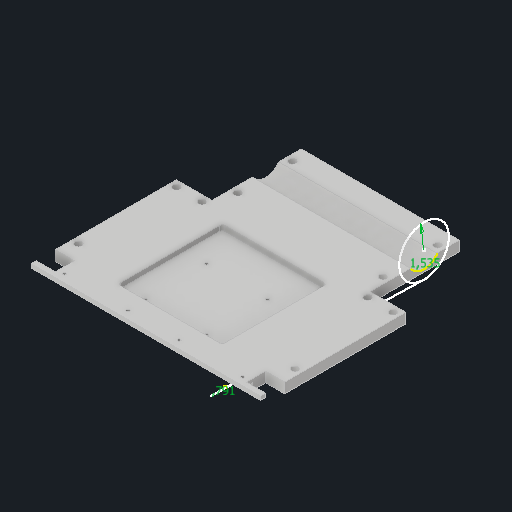
# Autodesk Inventor part: blacha
Saved by Autodesk Inventor 2023 (Build 270158000, 158)
## iProperties
Created: 2019-09-06
Part Number: blacha
Material: Generic
Document SubType Name: Modeling
Designer: Michal
Density: 1 g/cm^3
Appearance: Default
Author: Michal
Autodesk Inventor part; units mm, degrees
ref_plane "YZ Plane" through (0, 0, 0) normal (1, 0, 0) x (0, 1, 0)
ref_plane "XZ Plane" through (0, 0, 0) normal (0, 1, 0) x (-1, 0, 0)
ref_plane "XY Plane" through (0, 0, 0) normal (0, 0, 1) x (1, 0, 0)
sketch "Sketch1" plane through (0, 0, 0) normal (0, 1, 0) x (-1, 0, 0)
  line L0 (0, 0) -> (-180, 0)
  line L1 (0, 0) -> (0, -4)
  line L2 (0, -4) -> (-15, -4)
  line L3 (-15, -4) -> (-15, -19)
  line L4 (-15, -19) -> (0, -19)
  line L5 (-180, -4) -> (-165, -4)
  line L6 (-165, -4) -> (-165, -19)
  line L7 (-165, -19) -> (-180, -19)
  line L8 (-180, -4) -> (-180, 0)
  line L9 (0, -19) -> (0, -114)
  line L10 (0, -114) -> (-28, -114)
  line L11 (-28, -114) -> (-28, -184)
  line L12 (-28, -184) -> (-152, -184)
  line L13 (-152, -184) -> (-152, -114)
  line L14 (-152, -114) -> (-180, -114)
  line L15 (-180, -114) -> (-180, -19)
  dimension "d11" = 4
  dimension "d12" = 15
  dimension "d13" = 15
  dimension "d14" = 15
  dimension "d15" = 15
  dimension "d41" = 95
  dimension "d42" = 28
  dimension "d43" = 70
  dimension "d44" = 70
  dimension "d45" = 28
  constraints: 32 end point, 7 perpendicular, 3 horizontal, 2 parallel, 2 vertical
  measures "d11" distance of L0.start L1.end
  measures "d12" distance of L4.end L3.end
  measures "d13" distance of L3.end L2.end
  measures "d14" distance of L6.end L7.end
  measures "d15" distance of L5.end L6.end
  measures "d41" distance of L4.end L9.end
  measures "d42" distance of L9.end L10.end
  measures "d43" distance of L10.end L11.end
  measures "d44" distance of L12.end L13.end
  measures "d45" distance of L13.end L14.end
extrude "Extrusion1" add sketch "Sketch1" along normal blind 8
sketch "Sketch2" plane through (0, 0, 0) normal (0, -1, 0) x (1, 0, 0)
  line L0 (0, 0) -> (180, 0)
  line L1 (180, 0) -> (180, -9.1)
  line L2 (180, -9.1) -> (0, -9.1)
  line L3 (0, -9.1) -> (0, 0)
  dimension "d7" = 180
  dimension "d8" = 9.1
  constraints: 8 end point, 2 parallel, 1 horizontal, 1 perpendicular
  measures "d7" distance of L1.end L2.end
  measures "d8" distance of L0.end L1.end
extrude "Extrusion2" cut sketch "Sketch2" against normal blind 5
sketch "Sketch6" plane through (0, 5, 0) normal (0, -1, 0) x (1, 0, 0)
  line L0 (165, -9.1) -> (15, -9.1) projected
  line L1 (15, -9.1) -> (15, -6.1)
  line L2 (15, -19) -> (15, -4) projected
  line L3 (15, -6.1) -> (20, -6.1)
  line L4 (20, -6.1) -> (70, -6.1)
  line L5 (70, -6.1) -> (110, -6.1)
  line L6 (110, -6.1) -> (160, -6.1)
  point P0 (0, 0)
  dimension "d28" = 3
  dimension "d29" = 5
  dimension "d30" = 50
  dimension "d31" = 40
  dimension "d32" = 50
  constraints: 10 end point, 3 point on line, 1 parallel, 1 perpendicular
  measures "d28" distance of L0.end L1.end
  measures "d29" distance of L1.end L3.end
  measures "d30" distance of L3.end L4.end
  measures "d31" distance of L4.end L5.end
  measures "d32" distance of L5.end L6.end
hole "Hole1" at (20, 5, -6.1) at (70, 5, -6.1) at (110, 5, -6.1) at (160, 5, -6.1) direction (0, 1, 0) diameter 2.4638 end through all
sketch "Sketch7" plane through (152, 0, -114) normal (1, 0, 0) x (0, 0, -1)
  line L0 (70, 0) -> (42, 0)
  line L1 (70, 0) -> (0, 0) projected
  line L2 (42, 0) -> (42, 15)
  circle A0 centre (42, 15) radius 12.5
  point P0 (-114, 0)
  dimension "d46" = 28
  dimension "d47" = 15
  dimension "d48" = 25
  constraints: 4 end point, 1 centre point, 1 coincident, 1 point on line, 1 vertical
  measures "d46" distance of L0.start L0.end
  measures "d47" distance of L0.end L2.end
  measures "d48" diameter of A0
extrude "Extrusion5" cut sketch "Sketch7" against normal blind 124
sketch "Sketch8" plane through (0, 8, 0) normal (0, 1, 0) x (1, 0, 0)
  line L0 (0, 0) -> (180, 0) projected
  line L1 (0, 4) -> (0, 0) projected
  line L2 (0, 0) -> (48, 0)
  line L3 (48, 0) -> (48, 20)
  line L4 (48, 20) -> (130, 20)
  line L5 (130, 20) -> (130, 102)
  line L6 (130, 102) -> (48, 102)
  line L7 (48, 102) -> (48, 20)
  dimension "d114" = 48
  dimension "d115" = 20
  dimension "d116" = 82
  dimension "d117" = 82
  constraints: 12 end point, 2 parallel, 2 perpendicular, 1 horizontal, 1 point on line
  measures "d114" distance of L0.start L2.end
  measures "d115" distance of L2.end L3.end
  measures "d116" distance of L6.end L5.end
  measures "d117" distance of L5.end L4.end
extrude "Extrusion6" cut sketch "Sketch8" against normal blind 4
sketch "Sketch11" plane through (0, 0, 0) normal (0, -1, 0) x (1, 0, 0)
  line L0 (0, -114) -> (5, -114)
  line L1 (5, -114) -> (5, -109)
  line L2 (0, -109) -> (0, -114)
  line L3 (0, -109) -> (5, -109)
  line L4 (180, -114) -> (175, -114)
  line L5 (175, -114) -> (175, -109)
  line L6 (180, -109) -> (180, -114)
  line L7 (180, -109) -> (175, -109)
  line L8 (0, -19) -> (5, -19)
  line L9 (5, -19) -> (5, -32)
  line L10 (5, -32) -> (0, -32)
  line L11 (0, -32) -> (0, -19)
  line L12 (165, -19) -> (180, -19) projected
  line L13 (180, -19) -> (175, -19)
  line L14 (175, -19) -> (175, -32)
  line L15 (175, -32) -> (180, -32)
  line L16 (180, -32) -> (180, -19)
  line L17 (5, -109) -> (25, -109)
  line L18 (175, -109) -> (155, -109)
  line L19 (28, -184) -> (28, -114) projected
  line L20 (28, -184) -> (33, -184)
  line L21 (33, -184) -> (33, -172)
  line L22 (33, -172) -> (28, -172)
  line L23 (28, -172) -> (28, -184)
  line L24 (152, -184) -> (28, -184) projected
  line L25 (152, -184) -> (147, -184)
  line L26 (147, -184) -> (147, -172)
  line L27 (147, -172) -> (152, -172)
  line L28 (152, -172) -> (152, -184)
  line L29 (28, -145.6438) -> (28, -114) projected
  line L30 (28, -114) -> (33, -114)
  line L31 (33, -114) -> (33, -129)
  line L32 (33, -129) -> (28, -129)
  line L33 (28, -129) -> (28, -114)
  line L34 (180, -114) -> (152, -114) projected
  line L35 (152, -114) -> (147, -114)
  line L36 (147, -114) -> (147, -129)
  line L37 (147, -129) -> (152, -129)
  line L38 (152, -129) -> (152, -114)
  point P0 (0, 0)
  point P1 (145, -19)
  dimension "d88" = 5
  dimension "d89" = 5
  dimension "d92" = 5
  dimension "d105" = 5
  dimension "d106" = 13
  dimension "d107" = 20
  dimension "d108" = 20
  dimension "d131" = 5
  dimension "d132" = 12
  dimension "d133" = 5
  dimension "d134" = 12
  dimension "d136" = 5
  dimension "d137" = 15
  constraints: 68 end point, 14 parallel, 12 horizontal, 8 perpendicular
  measures "d88" distance of L2.start L1.end
  measures "d89" distance of L1.end L0.end
  measures "d92" distance of L5.end L6.start
  measures "d105" distance of L9.end L10.end
  measures "d106" distance of L8.end L9.end
  measures "d107" distance of L3.end L17.end
  measures "d108" distance of L7.end L18.end
  measures "d131" distance of L22.end L21.end
  measures "d132" distance of L21.end L20.end
  measures "d133" distance of L26.end L27.end
  measures "d134" distance of L25.end L26.end
  measures "d136" distance of L31.end L32.end
  measures "d137" distance of L30.end L31.end
hole "Hole4" at (5, 0, -109) at (175, 0, -109) at (175, 0, -32) at (5, 0, -32) at (155, 0, -109) at (25, 0, -109) at (33, 0, -129) at (33, 0, -172) at (147, 0, -172) at (147, 0, -129) direction (0, 1, 0) diameter 5.4 end through all countersink diameter 10.3886 countersink angle 90 clearance for "Countersunk Flat Head Screw ISO 2009/7046" size "M5" standard "ISO"
sketch "Sketch12" plane through (0, 4, 0) normal (0, 1, 0) x (1, 0, 0)
  line L0 (48, 20) -> (48, 102) projected
  line L1 (48, 20) -> (64.9, 20)
  line L2 (130, 20) -> (48, 20) projected
  line L3 (64.9, 20) -> (64.9, 24.4)
  line L4 (64.9, 24.4) -> (64.9, 72.6)
  line L5 (64.9, 24.4) -> (113.1, 24.4)
  line L6 (64.9, 24.4) -> (113.1, 72.6)
  point P0 (0, 0)
  dimension "d119" = 16.9
  dimension "d120" = 4.4
  dimension "d121" = 48.2
  dimension "d122" = 48.2
  constraints: 10 end point, 1 horizontal, 1 perpendicular, 1 point on line, 1 vertical
  measures "d119" distance of L0.start L1.end
  measures "d120" distance of L1.end L3.end
  measures "d121" distance of L3.end L4.end
  measures "d122" distance of L3.end L5.end
hole "Hole5" at (64.9, 4, -72.6) at (64.9, 4, -24.4) at (113.1, 4, -72.6) at (113.1, 4, -24.4) direction (0, -1, 0) diameter 2.4638 end through all
fillet "Fillet2" radius 2 4 edges at (48, 6, -102) (130, 6, -102) (130, 6, -20) (48, 6, -20)
sketch "Sketch13" plane through (152, 0, -184) normal (1, 0, 0) x (0, 0, -1)
  arc A0 (-38.3562, 8) -> (-17.6438, 8) centre (-28, 15) ccw projected
  circle A1 centre (-28, 15) radius 19.5
  line L0 (-174.9, 0) -> (-174.9, 5) projected
  line L1 (-174.9, 0) -> (-195, 0)
  line L2 (-195, 0) -> (-24.2057, -4.6095)
  point P0 (-184, 0)
  dimension "d138" = 39
  dimension "d139" = 20.1
  constraints: 4 end point, 1 centre point, 1 coincident, 1 horizontal, 1 tangent
  measures "d138" diameter of A1
  measures "d139" distance of L0.start L1.end
body "Solid1"
